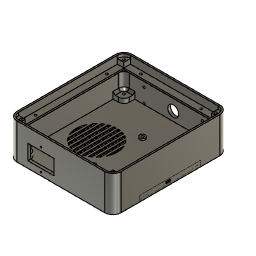
Solder Reflow Hot Plate Base (Autodesk Fusion 360 design; units mm, degrees)
Autodesk Fusion 360 part; units mm, degrees
note: some values were not read from the file. Chosen so that the rebuilt part matches the saved one: which bodies a step acts on; which face or edge a step refers to.
(part 1 of 2)
sketch "Base" plane through (0, 0, 0) normal (0, 0, 1) x (1, 0, 0) in component "Solder Reflow Hot Plate Base"
  line L0 (0, 0) -> (190, 0)
  line L1 (190, 0) -> (190, 210)
  line L2 (190, 210) -> (0, 210)
  line L3 (0, 210) -> (0, 0)
  dimension "d1" = 190
  dimension "d2" = 210
  constraint horizontal L0
  constraint vertical L1
  constraint horizontal L2
  constraint vertical L3
  constraint coincident L0.start L3.end
  measures "d1" distance of L0.start L0.end
  measures "d2" distance of L0.start L2.end
extrude "Extrude1" add sketch "Base" along normal blind 65 makes body 1 in component "Solder Reflow Hot Plate Base"
fillet "Fillet1" radius 15 4 edges at (0, 210, 32.5) (0, 0, 32.5) (190, 0, 32.5) (190, 210, 32.5) on bodies 1 in component "Solder Reflow Hot Plate Base"
shell "Shell1" thickness 5 removed faces 1 at (63.3333, 135, 65) on bodies 1 in component "Solder Reflow Hot Plate Base"
extrude "Extrude2" cut 1 faces at (65, 135, 5) along direction (0, 0, -1) blind 3 on bodies 1 bodies 1 in component "Solder Reflow Hot Plate Base"
sketch "Board Mount Split Sketch" plane through (0, 0, 2) normal (0, 0, 1) x (-1, 0, 0) in component "Solder Reflow Hot Plate Base"
  arc A0 (-185, -195) -> (-175, -205) centre (-175, -195) ccw
  line L0 (-175, -205) -> (-15, -205)
  arc A1 (-15, -205) -> (-5, -195) centre (-15, -195) ccw
  line L1 (-5, -195) -> (-5, -15)
  arc A2 (-5, -15) -> (-15, -5) centre (-15, -15) ccw
  line L2 (-15, -5) -> (-175, -5)
  arc A3 (-175, -5) -> (-185, -15) centre (-175, -15) ccw
  line L3 (-185, -15) -> (-185, -195)
  line L4 (-184.6, -15) -> (-184.6, -195)
  arc A4 (-184.6, -195) -> (-175, -204.6) centre (-175, -195) ccw
  line L5 (-175, -204.6) -> (-15, -204.6)
  arc A5 (-15, -204.6) -> (-5.4, -195) centre (-15, -195) ccw
  line L6 (-5.4, -195) -> (-5.4, -15)
  arc A6 (-5.4, -15) -> (-15, -5.4) centre (-15, -15) ccw
  line L7 (-15, -5.4) -> (-175, -5.4)
  arc A7 (-175, -5.4) -> (-184.6, -15) centre (-175, -15) ccw
  line L8 (-185, -15) -> (-185, -195)
  arc A8 (-185, -195) -> (-175, -205) centre (-175, -195) ccw
  line L9 (-175, -205) -> (-15, -205)
  arc A9 (-15, -205) -> (-5, -195) centre (-15, -195) ccw
  line L10 (-5, -195) -> (-5, -15)
  arc A10 (-5, -15) -> (-15, -5) centre (-15, -15) ccw
  line L11 (-15, -5) -> (-175, -5)
  arc A11 (-175, -5) -> (-185, -15) centre (-175, -15) ccw
  dimension "d10" = -0.4
  dimension "d11" = 0
  measures "d11" distance of L3
sketch "Sketch1" plane through (0, 0, 2) normal (0, 0, 1) x (-1, 0, 0)
  arc A0 (-185, -195) -> (-175, -205) centre (-175, -195) ccw
  line L0 (-175, -205) -> (-15, -205)
  arc A1 (-15, -205) -> (-5, -195) centre (-15, -195) ccw
  line L1 (-5, -195) -> (-5, -15)
  arc A2 (-5, -15) -> (-15, -5) centre (-15, -15) ccw
  line L2 (-15, -5) -> (-175, -5)
  arc A3 (-175, -5) -> (-185, -15) centre (-175, -15) ccw
  line L3 (-185, -15) -> (-185, -195)
  line L4 (-5, -195) -> (-5, -15)
  arc A4 (-5, -15) -> (-15, -5) centre (-15, -15) ccw
  line L5 (-15, -5) -> (-175, -5)
  arc A5 (-175, -5) -> (-185, -15) centre (-175, -15) ccw
  line L6 (-185, -15) -> (-185, -195)
  arc A6 (-185, -195) -> (-175, -205) centre (-175, -195) ccw
  line L7 (-175, -205) -> (-15, -205)
  arc A7 (-15, -205) -> (-5, -195) centre (-15, -195) ccw
  dimension "d12" = 0
  measures "d12" distance of L1
split "Split2" by curves path "Sketch1" along L4 A4 L5 A5 L6 A6 L7 A7 bodies 1 makes body 2 at (0, 135, 21.6667) in component "Solder Reflow Hot Plate Base"
sketch "Sketch2" plane through (0, 0, 2) normal (0, 0, 1) x (-1, 0, 0)
  arc A0 (-185, -195) -> (-175, -205) centre (-175, -195) ccw
  line L0 (-175, -205) -> (-15, -205)
  arc A1 (-15, -205) -> (-5, -195) centre (-15, -195) ccw
  line L1 (-5, -195) -> (-5, -15)
  arc A2 (-5, -15) -> (-15, -5) centre (-15, -15) ccw
  line L2 (-15, -5) -> (-175, -5)
  arc A3 (-175, -5) -> (-185, -15) centre (-175, -15) ccw
  line L3 (-185, -15) -> (-185, -195)
  line L4 (-5.4, -195) -> (-5.4, -15)
  arc A4 (-5.4, -15) -> (-15, -5.4) centre (-15, -15) ccw
  line L5 (-15, -5.4) -> (-175, -5.4)
  arc A5 (-175, -5.4) -> (-184.6, -15) centre (-175, -15) ccw
  line L6 (-184.6, -15) -> (-184.6, -195)
  arc A6 (-184.6, -195) -> (-175, -204.6) centre (-175, -195) ccw
  line L7 (-175, -204.6) -> (-15, -204.6)
  arc A7 (-15, -204.6) -> (-5.4, -195) centre (-15, -195) ccw
  dimension "d13" = -0.4
extrude "Extrude3" cut sketch "Sketch2" against normal up to surface (2 mm away) bodies 1 in component "Solder Reflow Hot Plate Base"
ref_plane "WorkPlane1" through (95, 105, 0) normal (0, 0, -1) x (-1, 0, 0) in component "Solder Reflow Hot Plate Base"
sketch "Sketch5" plane through (0, 0, 2) normal (0, 0, 1) x (-1, 0, 0) in component "Solder Reflow Hot Plate Base"
  line L0 (-15, -5.4) -> (-175, -5.4)
  arc A0 (-175, -5.4) -> (-184.6, -15) centre (-175, -15) ccw
  line L1 (-184.6, -15) -> (-184.6, -195)
  arc A1 (-184.6, -195) -> (-175, -204.6) centre (-175, -195) ccw
  line L2 (-175, -204.6) -> (-15, -204.6)
  arc A2 (-15, -204.6) -> (-5.4, -195) centre (-15, -195) ccw
  line L3 (-5.4, -195) -> (-5.4, -15)
  arc A3 (-5.4, -15) -> (-15, -5.4) centre (-15, -15) ccw
  line L4 (-184.6, -105) -> (-5.4, -105) construction
  line L5 (-184.6, -105) -> (-184.6, -50) construction
  line L6 (-184.6, -105) -> (-184.6, -160) construction
  line L7 (-184.6, -50) -> (-188.8, -50)
  line L8 (-184.6, -160) -> (-188.8, -160)
  line L9 (-188.8, -160) -> (-188.8, -50)
  line L10 (-184.6, -50) -> (-184.6, -160)
  dimension "d18" = 55
  dimension "d19" = 55
  dimension "d20" = 4.2
  dimension "d21" = 4.2
  constraint midpoint L1 L4.start
  constraint midpoint L3 L4.end
  constraint perpendicular L4 L5
  constraint perpendicular L4 L6
  constraint perpendicular L1 L7
  constraint perpendicular L1 L8
  measures "d18" distance of L4.start L5.end
  measures "d19" distance of L4.start L6.end
  measures "d20" distance of L5.end L7.end
  measures "d21" distance of L6.end L8.end
extrude "Extrude4" add sketch "Sketch5" against normal up to surface (2 mm away) contours L1 L7 L8 L9 L10 bodies 1 in component "Solder Reflow Hot Plate Base"
sketch "Sketch6" plane through (0, 0, 0) normal (0, 0, -1) x (1, 0, 0) in component "Solder Reflow Hot Plate Base"
  line L0 (175, -205) -> (15, -205)
  arc A0 (5, -195) -> (15, -205) centre (15, -195) ccw
  line L1 (5, -195) -> (5, -15)
  arc A1 (15, -5) -> (5, -15) centre (15, -15) ccw
  line L2 (15, -5) -> (175, -5)
  arc A2 (185, -15) -> (175, -5) centre (175, -15) ccw
  line L3 (185, -15) -> (185, -195)
  arc A3 (175, -205) -> (185, -195) centre (175, -195) ccw
  arc A4 (175, -210) -> (190, -195) centre (175, -195) ccw
  line L4 (190, -195) -> (190, -15)
  arc A5 (190, -15) -> (175, 0) centre (175, -15) ccw
  line L5 (175, 0) -> (15, 0)
  arc A6 (15, 0) -> (0, -15) centre (15, -15) ccw
  line L6 (0, -15) -> (0, -195)
  arc A7 (0, -195) -> (15, -210) centre (15, -195) ccw
  line L7 (15, -210) -> (175, -210)
  line L8 (190, -105) -> (189, -105) construction
  line L9 (189, -105) -> (189, -160.4)
  line L10 (189, -105) -> (189, -49.6)
  line L11 (189, -160.4) -> (185, -160.4)
  line L12 (189, -49.6) -> (185, -49.6)
  line L13 (185, -49.6) -> (185, -160.4)
  dimension "d27" = 55.4
  dimension "d28" = 55.4
  dimension "d31" = 1
  constraint midpoint L4 L8.start
  constraint perpendicular L4 L8
  constraint perpendicular L8 L9
  constraint perpendicular L8 L10
  constraint coincident L3 L11.end
  constraint perpendicular L3 L11
  constraint coincident L3 L12.end
  constraint perpendicular L3 L12
  measures "d27" distance of L8.end L9.end
  measures "d28" distance of L8.end L10.end
  measures "d31" distance of L4 L10
extrude "Extrude5" cut sketch "Sketch6" against normal blind 10 contours L3 L9 L10 L11 L12 L13 bodies 2 in component "Solder Reflow Hot Plate Base"
sketch "Sketch7" plane through (0, 0, 2) normal (0, 0, 1) x (-1, 0, 0) in component "Solder Reflow Hot Plate Base"
  line L0 (-15, -5.4) -> (-175, -5.4)
  arc A0 (-175, -5.4) -> (-184.6, -15) centre (-175, -15) ccw
  line L1 (-184.6, -15) -> (-184.6, -50)
  line L2 (-184.6, -50) -> (-188.8, -50)
  line L3 (-188.8, -50) -> (-188.8, -160)
  line L4 (-188.8, -160) -> (-184.6, -160)
  line L5 (-184.6, -160) -> (-184.6, -195)
  arc A1 (-184.6, -195) -> (-175, -204.6) centre (-175, -195) ccw
  line L6 (-175, -204.6) -> (-15, -204.6)
  arc A2 (-15, -204.6) -> (-5.4, -195) centre (-15, -195) ccw
  line L7 (-5.4, -195) -> (-5.4, -15)
  arc A3 (-5.4, -15) -> (-15, -5.4) centre (-15, -15) ccw
  line L8 (-188.8, -105) -> (-5.4, -105) construction
  line L9 (-184, -105) -> (-184, -60) construction
  line L10 (-184, -105) -> (-184, -150) construction
  circle A4 centre (-184, -60) radius 2.05
  circle A5 centre (-184, -150) radius 2.05
  line L11 (-94, -105) -> (-94, -60) construction
  line L12 (-94, -105) -> (-94, -150) construction
  circle A6 centre (-94, -60) radius 2.05
  circle A7 centre (-94, -150) radius 2.05
  circle A8 centre (-94, -150) radius 5
  circle A9 centre (-94, -60) radius 5
  line L13 (-184, -55) -> (-188.8, -55)
  line L14 (-184, -65) -> (-188.8, -65)
  arc A10 (-184, -65) -> (-184, -55) centre (-184, -60) ccw
  line L15 (-188.8, -55) -> (-188.8, -65)
  line L16 (-184, -145) -> (-188.8, -145)
  line L17 (-184, -155) -> (-188.8, -155)
  arc A11 (-184, -155) -> (-184, -145) centre (-184, -150) ccw
  line L18 (-188.8, -145) -> (-188.8, -155)
  dimension "d32" = 45
  dimension "d33" = 45
  dimension "d34" = 4.8
  dimension "d35" = 4.1
  dimension "d36" = 4.1
  dimension "d37" = 45
  dimension "d38" = 45
  dimension "d39" = 90
  dimension "d40" = 4.1
  dimension "d41" = 4.1
  dimension "d42" = 10
  dimension "d43" = 10
  dimension "d44" = 10
  dimension "d45" = 10
  constraint midpoint L3 L8.start
  constraint midpoint L7 L8.end
  constraint coincident L8 L9.start
  constraint perpendicular L8 L9
  constraint perpendicular L8 L10
  constraint coincident L9.end A4.centre
  constraint coincident L10.end A5.centre
  constraint coincident L8 L11.start
  constraint perpendicular L8 L11
  constraint perpendicular L8 L12
  constraint coincident L11.end A6.centre
  constraint coincident L12.end A7.centre
  constraint coincident L3 L13.end
  constraint tangent L13 A10
  constraint perpendicular L3 L13
  constraint coincident L9 L14.start
  constraint coincident L3 L14.end
  constraint tangent L14 A10
  constraint coincident L10 L16.start
  constraint coincident L3 L16.end
  constraint tangent L16 A11
  constraint coincident L3 L17.end
  constraint tangent L17 A11
  constraint perpendicular L3 L17
  measures "d32" distance of L9.start L9.end
  measures "d33" distance of L9.start L10.end
  measures "d34" distance of L3 L9
  measures "d35" diameter of A4
  measures "d36" diameter of A5
  measures "d37" distance of L11.start L11.end
  measures "d38" distance of L11.start L12.end
  measures "d39" distance of L9 L11
  measures "d40" diameter of A6
  measures "d41" diameter of A7
  measures "d42" diameter of A8
  measures "d43" diameter of A9
  measures "d44" diameter of A10
  measures "d45" diameter of A11
extrude "Extrude6" add sketch "Sketch7" along normal blind 3 contours L3 L13 L14 A10 L15 | L3 L16 L17 A11 L18 | A8 | A9 bodies 1 in component "Solder Reflow Hot Plate Base"
extrude "Extrude7" cut 4 faces at (94.4261, 150.7379, 2) (184.6757, 149.8982, 2) (93.7504, 60.6361, 2) (183.4991, 59.1324, 2) along direction (0, 0, 1) up to surface end surface through (0, 0, 0) normal (0, 0, -1) offset 0 on bodies 1 bodies 1 in component "Solder Reflow Hot Plate Base"
sketch "Sketch8" plane through (190, 0, 0) normal (1, 0, 0) x (0, 1, 0) in component "Solder Reflow Hot Plate Base"
  line L0 (195, 0) -> (195, 65)
  line L1 (195, 65) -> (15, 65)
  line L2 (15, 65) -> (15, 0)
  line L3 (15, 0) -> (195, 0)
  line L4 (105, 0) -> (105, 65) construction
  line L5 (100.8, 0) -> (100.8, 65) construction
  line L6 (55, 5) -> (65, 5) construction
  line L7 (145, 5) -> (155, 5) construction
  line L8 (55, 5) -> (155, 5) construction
  line L9 (55, 4.8) -> (155, 4.8) construction
  line L10 (96.8, 0) -> (96.8, 65) construction
  line L11 (104.8, 0) -> (104.8, 65) construction
  line L12 (15, 8.2) -> (195, 8.2) construction
  line L13 (96.8, 8.2) -> (104.8, 8.2)
  line L14 (104.8, 8.2) -> (104.8, 4.8)
  line L15 (104.8, 4.8) -> (96.8, 4.8)
  line L16 (96.8, 4.8) -> (96.8, 8.2)
  dimension "d50" = 4.2
  dimension "d51" = 0.2
  dimension "d52" = 4
  dimension "d53" = 4
  dimension "d54" = 3.4
  constraint midpoint L3 L4.start
  constraint midpoint L1 L4.end
  constraint coincident L3 L5.start
  constraint coincident L1 L5.end
  constraint perpendicular L1 L5
  constraint coincident L6.start L8.start
  constraint coincident L7.end L8.end
  constraint parallel L8 L9
  constraint coincident L3 L10.start
  constraint coincident L1 L10.end
  constraint perpendicular L1 L10
  constraint coincident L3 L11.start
  constraint coincident L1 L11.end
  constraint perpendicular L1 L11
  constraint coincident L2 L12.start
  constraint coincident L0 L12.end
  constraint perpendicular L0 L12
  constraint horizontal L13
  constraint vertical L14
  constraint horizontal L15
  constraint vertical L16
  constraint coincident L9 L14.end
  constraint coincident L11 L14.end
  constraint coincident L12 L13.start
  constraint coincident L10 L13.start
  measures "d50" distance of L4 L5
  measures "d51" distance of L8 L9
  measures "d52" distance of L5 L10
  measures "d53" distance of L5 L11
  measures "d54" distance of L9 L12
extrude "Extrude8" cut sketch "Sketch8" against normal up to surface (1 mm away) contours L13 L14 L15 L16 bodies 2 in component "Solder Reflow Hot Plate Base"
chamfer "Chamfer1" distance 0.5 angle 45 2 edges at (189.5, 104.8, 4.8) (189.5, 96.8, 4.8) on bodies 2 in component "Solder Reflow Hot Plate Base"
ref_plane "WorkPlane2" through (95, 105, 2) normal (0, 0, -1) x (-1, 0, 0) in component "Solder Reflow Hot Plate Base"
sketch "Sketch9" plane through (95, 105, 2) normal (0, 0, -1) x (1, 0, 0) in component "Solder Reflow Hot Plate Base"
  line L0 (90, -90) -> (90, 90) construction
  arc A0 (90, 90) -> (80, 100) centre (80, 90) ccw construction
  line L1 (80, 100) -> (-80, 100) construction
  arc A1 (-80, 100) -> (-90, 90) centre (-80, 90) ccw construction
  line L2 (-90, 90) -> (-90, -90) construction
  arc A2 (-90, -90) -> (-80, -100) centre (-80, -90) ccw construction
  line L3 (-80, -100) -> (80, -100) construction
  arc A3 (80, -100) -> (90, -90) centre (80, -90) ccw construction
  arc A4 (80, -100) -> (90, -90) centre (80, -90) ccw construction
  line L4 (90, -90) -> (90, 90) construction
  arc A5 (90, 90) -> (80, 100) centre (80, 90) ccw construction
  line L5 (80, 100) -> (-80, 100) construction
  arc A6 (-80, 100) -> (-90, 90) centre (-80, 90) ccw construction
  line L6 (-90, 90) -> (-90, -90) construction
  arc A7 (-90, -90) -> (-80, -100) centre (-80, -90) ccw construction
  line L7 (-80, -100) -> (80, -100) construction
  arc A8 (80, -105) -> (95, -90) centre (80, -90) ccw construction
  line L8 (80, -105) -> (-80, -105) construction
  arc A9 (-95, -90) -> (-80, -105) centre (-80, -90) ccw construction
  line L9 (-95, -90) -> (-95, 90) construction
  arc A10 (-80, 105) -> (-95, 90) centre (-80, 90) ccw construction
  line L10 (-80, 105) -> (80, 105) construction
  arc A11 (95, 90) -> (80, 105) centre (80, 90) ccw construction
  line L11 (95, 90) -> (95, -90) construction
  line L12 (80, 100) -> (80, -100) construction
  line L13 (90, -90) -> (-90, -90) construction
  line L14 (-80, -100) -> (-80, 100) construction
  line L15 (90, 90) -> (-90, 90) construction
  circle A12 centre (80, 90) radius 2.05
  line L16 (80, 80) -> (90, 80)
  line L17 (70, 90) -> (70, 100)
  line L18 (70, 100) -> (80, 100)
  line L19 (90, 80) -> (90, 90)
  arc A13 (70, 90) -> (80, 80) centre (80, 90) ccw
  arc A14 (90, 90) -> (80, 100) centre (80, 90) ccw
  line L20 (0, 100) -> (0, -100) construction
  line L21 (90, 0) -> (-90, 0) construction
  line L22 (-70, 100) -> (-80, 100)
  line L23 (-70, 90) -> (-70, 100)
  arc A15 (-80, 80) -> (-70, 90) centre (-80, 90) ccw
  line L24 (-80, 80) -> (-90, 80)
  line L25 (-90, 80) -> (-90, 90)
  arc A16 (-80, 100) -> (-90, 90) centre (-80, 90) ccw
  circle A17 centre (-80, 90) radius 2.05
  line L26 (80, -80) -> (90, -80)
  line L27 (90, -80) -> (90, -90)
  arc A18 (80, -100) -> (90, -90) centre (80, -90) ccw
  line L28 (70, -100) -> (80, -100)
  line L29 (70, -90) -> (70, -100)
  arc A19 (80, -80) -> (70, -90) centre (80, -90) ccw
  circle A20 centre (80, -90) radius 2.05
  line L30 (-70, -90) -> (-70, -100)
  line L31 (-70, -100) -> (-80, -100)
  arc A21 (-90, -90) -> (-80, -100) centre (-80, -90) ccw
  line L32 (-90, -80) -> (-90, -90)
  line L33 (-80, -80) -> (-90, -80)
  arc A22 (-70, -90) -> (-80, -80) centre (-80, -90) ccw
  circle A23 centre (-80, -90) radius 2.05
  dimension "d60" = 4.1
  constraint coincident A0.end L1.start
  constraint coincident L3.end A3.start
  constraint coincident L0.start A3.end
  constraint coincident L2.end A2.start
  constraint coincident A2.end L3.start
  constraint coincident L1.end A1.start
  constraint coincident L0.end A0.start
  constraint coincident A1.end L2.start
  constraint concentric A0 A12
  constraint concentric A5 A13
  constraint coincident A0.end A13
  constraint coincident L12 L16.start
  constraint coincident L4 L16.end
  constraint tangent L16 A13
  constraint coincident L15 L17.start
  constraint coincident L1 L17.end
  constraint tangent L17 A13
  constraint concentric A13 A14
  constraint midpoint L5 L20.start
  constraint midpoint L3 L20.end
  constraint midpoint L0 L21.start
  constraint midpoint L6 L21.end
  constraint symmetric L0.end L20 A1.end
  constraint symmetric A0.end L20 L1.end
  constraint symmetric A12 L20 A17
  constraint symmetric L16.start L20 A15.start
  constraint symmetric L16.end L20 L24.end
  constraint symmetric L17.start L20 L23.start
  constraint symmetric L17.end L20 L22.start
  constraint symmetric A13 L20 A15
  constraint symmetric A14 L20 A16
  constraint symmetric L0.end L21 L0.start
  constraint symmetric A0.end L21 L3.end
  constraint symmetric A12 L21 A20
  constraint symmetric L16.start L21 L26.start
  constraint symmetric L16.end L21 L26.end
  constraint symmetric L17.start L21 L29.start
  constraint symmetric L17.end L21 L28.start
  constraint symmetric A13 L21 A19
  constraint symmetric A14 L21 A18
  constraint symmetric L21 L22.start L30.end
  constraint symmetric L21 L1.end A2.end
  constraint symmetric L21 L23.start L30.start
  constraint symmetric L21 A15.start L33.start
  constraint symmetric L21 A15 A22
  constraint symmetric L21 L24.end L32.start
  constraint symmetric L21 A1.end L2.end
  constraint symmetric L21 A16 A21
  constraint symmetric L21 A17 A23
  measures "d60" diameter of A12
extrude "Extrude9" add sketch "Sketch9" against normal blind 8 bodies 2 in component "Solder Reflow Hot Plate Base"
chamfer "Chamfer2" distance 4 angle 45 12 edges at (182.0711, 7.9289, 10) (170, 5, 10) (185, 20, 10) (20, 5, 10) (7.9289, 7.9289, 10) (5, 20, 10) (20, 205, 10) (5, 190, 10) (7.9289, 202.0711, 10) (170, 205, 10) (182.0711, 202.0711, 10) (185, 190, 10) on bodies 2 in component "Solder Reflow Hot Plate Base"
sketch "Sketch10" plane through (0, 0, 0) normal (0, 0, -1) x (1, 0, 0) in component "Solder Reflow Hot Plate Base"
  circle A0 centre (94, -60) radius 2.05
  circle A1 centre (94, -150) radius 2.05
  circle A2 centre (184, -150) radius 2.05
  circle A3 centre (184, -60) radius 2.05
  line L0 (175, -5.4) -> (15, -5.4)
  arc A4 (15, -5.4) -> (5.4, -15) centre (15, -15) ccw
  line L1 (5.4, -15) -> (5.4, -195)
  arc A5 (5.4, -195) -> (15, -204.6) centre (15, -195) ccw
  line L2 (15, -204.6) -> (175, -204.6)
  arc A6 (175, -204.6) -> (184.6, -195) centre (175, -195) ccw
  line L3 (184.6, -195) -> (184.6, -160)
  line L4 (184.6, -160) -> (188.8, -160)
  line L5 (188.8, -160) -> (188.8, -50)
  line L6 (188.8, -50) -> (184.6, -50)
  line L7 (184.6, -50) -> (184.6, -15)
  arc A7 (184.6, -15) -> (175, -5.4) centre (175, -15) ccw
  circle A8 centre (175, -15) radius 2.05
  circle A9 centre (15, -15) radius 2.05
  circle A10 centre (15, -195) radius 2.05
  circle A11 centre (175, -195) radius 2.05
  circle A12 centre (15, -195) radius 1.9
  circle A13 centre (175, -195) radius 1.9
  circle A14 centre (175, -15) radius 1.9
  circle A15 centre (15, -15) radius 1.9
  dimension "d71" = 3.8
  dimension "d72" = 3.8
  dimension "d73" = 3.8
  dimension "d74" = 3.8
  constraint concentric A10 A12
  constraint concentric A11 A13
  constraint concentric A7 A14
  constraint concentric A9 A15
  measures "d71" diameter of A12
  measures "d72" diameter of A13
  measures "d73" diameter of A14
  measures "d74" diameter of A15
extrude "Extrude10" cut sketch "Sketch10" against normal up to surface (2 mm away) contours A12 | A13 | A14 | A15 bodies 1 in component "Solder Reflow Hot Plate Base"
ref_plane "WorkPlane3" through (95, 105, 31) normal (0, 0, -1) x (-1, 0, 0) in component "Solder Reflow Hot Plate Base"
ref_plane "WorkPlane4" through (95, 105, 60) normal (0, 0, 1) x (1, 0, 0) in component "Solder Reflow Hot Plate Base"
ref_plane "WorkPlane5" through (95, 105, 51) normal (0, 0, 1) x (1, 0, 0) in component "Solder Reflow Hot Plate Base"
sketch "Sketch11" plane through (0, 0, 65) normal (0, 0, 1) x (-1, 0, 0) in component "Solder Reflow Hot Plate Base"
  arc A0 (-185, -195) -> (-175, -205) centre (-175, -195) ccw
  line L0 (-185, -195) -> (-185, -15)
  arc A1 (-175, -5) -> (-185, -15) centre (-175, -15) ccw
  line L1 (-175, -5) -> (-15, -5)
  arc A2 (-5, -15) -> (-15, -5) centre (-15, -15) ccw
  line L2 (-5, -15) -> (-5, -195)
  arc A3 (-15, -205) -> (-5, -195) centre (-15, -195) ccw
  line L3 (-15, -205) -> (-175, -205)
  arc A4 (-190, -195) -> (-175, -210) centre (-175, -195) ccw
  line L4 (-175, -210) -> (-15, -210)
  arc A5 (-15, -210) -> (0, -195) centre (-15, -195) ccw
  line L5 (0, -195) -> (0, -15)
  arc A6 (0, -15) -> (-15, 0) centre (-15, -15) ccw
  line L6 (-15, 0) -> (-175, 0)
  arc A7 (-175, 0) -> (-190, -15) centre (-175, -15) ccw
  line L7 (-190, -15) -> (-190, -195)
  arc A8 (-3, -15) -> (-15, -3) centre (-15, -15) ccw
  line L8 (-175, -3) -> (-15, -3)
  arc A9 (-175, -3) -> (-187, -15) centre (-175, -15) ccw
  line L9 (-187, -195) -> (-187, -15)
  arc A10 (-187, -195) -> (-175, -207) centre (-175, -195) ccw
  line L10 (-15, -207) -> (-175, -207)
  arc A11 (-15, -207) -> (-3, -195) centre (-15, -195) ccw
  line L11 (-3, -15) -> (-3, -195)
  arc A12 (-5, -15) -> (-15, -5) centre (-15, -15) ccw
  line L12 (-175, -5) -> (-15, -5)
  arc A13 (-175, -5) -> (-185, -15) centre (-175, -15) ccw
  line L13 (-185, -195) -> (-185, -15)
  arc A14 (-185, -195) -> (-175, -205) centre (-175, -195) ccw
  line L14 (-15, -205) -> (-175, -205)
  arc A15 (-15, -205) -> (-5, -195) centre (-15, -195) ccw
  line L15 (-5, -15) -> (-5, -195)
  dimension "d80" = -2
  dimension "d81" = 0
extrude "Extrude11" cut sketch "Sketch11" against normal up to surface (14 mm away) contours A8 L8 A9 L9 A10 L10 A11 L11 bodies 2 in component "Solder Reflow Hot Plate Base"
sketch "Sketch12" plane through (0, 0, 51) normal (0, 0, 1) x (-1, 0, 0) in component "Solder Reflow Hot Plate Base"
  line L0 (-175, -5) -> (-15, -5)
  arc A0 (-5, -15) -> (-15, -5) centre (-15, -15) ccw
  line L1 (-5, -15) -> (-5, -195)
  arc A1 (-15, -205) -> (-5, -195) centre (-15, -195) ccw
  line L2 (-15, -205) -> (-175, -205)
  arc A2 (-185, -195) -> (-175, -205) centre (-175, -195) ccw
  line L3 (-185, -195) -> (-185, -15)
  arc A3 (-175, -5) -> (-185, -15) centre (-175, -15) ccw
  line L4 (-187, -15) -> (-187, -195)
  arc A4 (-187, -195) -> (-175, -207) centre (-175, -195) ccw
  line L5 (-175, -207) -> (-15, -207)
  arc A5 (-15, -207) -> (-3, -195) centre (-15, -195) ccw
  line L6 (-3, -195) -> (-3, -15)
  arc A6 (-3, -15) -> (-15, -3) centre (-15, -15) ccw
  line L7 (-15, -3) -> (-175, -3)
  arc A7 (-175, -3) -> (-187, -15) centre (-175, -15) ccw
  line L8 (-185, -15) -> (-5, -15) construction
  line L9 (-175, -5) -> (-175, -205) construction
  line L10 (-175, -15) -> (-15, -15)
  line L11 (-175, -195) -> (-175, -15)
  line L12 (-15, -195) -> (-175, -195)
  line L13 (-15, -15) -> (-15, -195)
  dimension "d84" = 10
  constraint coincident L3.end A3.end
  constraint coincident A0.start L1.start
  constraint coincident L0.start A3.start
  constraint coincident L2.end A2.end
extrude "Extrude12" add sketch "Sketch12" against normal blind 3 contours L0 A0 L1 A1 L2 A2 L3 A3 bodies 2 in component "Solder Reflow Hot Plate Base"
chamfer "Chamfer3" distance 9.8 angle 45 8 edges at (185, 105, 48) (182.0711, 202.0711, 48) (95, 205, 48) (7.9289, 202.0711, 48) (5, 105, 48) (7.9289, 7.9289, 48) (95, 5, 48) (182.0711, 7.9289, 48) on bodies 2 in component "Solder Reflow Hot Plate Base"
sketch "Sketch13" plane through (0, 0, 51) normal (0, 0, 1) x (-1, 0, 0) in component "Solder Reflow Hot Plate Base"
  line L0 (-175, -15) -> (-15, -15)
  line L1 (-15, -15) -> (-15, -195)
  line L2 (-15, -195) -> (-175, -195)
  line L3 (-175, -195) -> (-175, -15)
  line L4 (-187, -15) -> (-187, -195)
  arc A0 (-187, -195) -> (-175, -207) centre (-175, -195) ccw
  line L5 (-175, -207) -> (-15, -207)
  arc A1 (-15, -207) -> (-3, -195) centre (-15, -195) ccw
  line L6 (-3, -195) -> (-3, -15)
  arc A2 (-3, -15) -> (-15, -3) centre (-15, -15) ccw
  line L7 (-15, -3) -> (-175, -3)
  arc A3 (-175, -3) -> (-187, -15) centre (-175, -15) ccw
  line L8 (-187, -15) -> (-3, -15) construction
  line L9 (-175, -3) -> (-175, -207) construction
  line L10 (-186.619, -12) -> (-3.381, -12) construction
  line L11 (-178, -3.381) -> (-178, -206.619) construction
  circle A4 centre (-178, -12) radius 2.05
  line L12 (-95, -3) -> (-95, -207) construction
  line L13 (-187, -105) -> (-3, -105) construction
  circle A5 centre (-12, -12) radius 2.05
  circle A6 centre (-12, -198) radius 2.05
  circle A7 centre (-178, -198) radius 2.05
  dimension "d88" = 3
  dimension "d89" = 3
  dimension "d90" = 4.1
  constraint coincident L4.start A3.end
  constraint coincident L6.end A2.start
  constraint coincident L7.end A3.start
  constraint coincident A0.end L5.start
  constraint horizontal L10
  constraint coincident A3 L10.start
  constraint coincident A2 L10.end
  constraint vertical L11
  constraint coincident A3 L11.start
  constraint coincident A0 L11.end
  constraint coincident L11 A4.centre
  constraint coincident L10 A4.centre
  constraint midpoint L7 L12.start
  constraint midpoint L5 L12.end
  constraint midpoint L4 L13.start
  constraint midpoint L6 L13.end
  constraint symmetric A4 L12 A5
  constraint symmetric A4 L13 A7
  constraint symmetric L13 A5 A6
  measures "d88" distance of L8 L10
  measures "d89" distance of L9 L11
  measures "d90" diameter of A4
sketch "Sketch15" plane through (0, 0, 51) normal (0, 0, 1) x (-1, 0, 0) in component "Solder Reflow Hot Plate Base"
  line L0 (-175, -15) -> (-15, -15)
  line L1 (-15, -15) -> (-15, -195)
  line L2 (-15, -195) -> (-175, -195)
  line L3 (-175, -195) -> (-175, -15)
  line L4 (-187, -15) -> (-187, -195)
  arc A0 (-187, -195) -> (-175, -207) centre (-175, -195) ccw
  line L5 (-175, -207) -> (-15, -207)
  arc A1 (-15, -207) -> (-3, -195) centre (-15, -195) ccw
  line L6 (-3, -195) -> (-3, -15)
  arc A2 (-3, -15) -> (-15, -3) centre (-15, -15) ccw
  line L7 (-15, -3) -> (-175, -3)
  arc A3 (-175, -3) -> (-187, -15) centre (-175, -15) ccw
  line L8 (-165, -15) -> (-165, -5)
  line L9 (-175, -25) -> (-185, -25)
  arc A4 (-175, -3) -> (-187, -15) centre (-175, -15) ccw
  line L10 (-95, -3) -> (-95, -207) construction
  line L11 (-187, -105) -> (-3, -105) construction
  line L12 (-175, -15) -> (-175, -14)
  line L13 (-175, -14) -> (-175, -3)
  line L14 (-175, -15) -> (-187, -15)
  line L15 (-15, -15) -> (-3, -15)
  line L16 (-15, -195) -> (-3, -195)
  line L17 (-175, -195) -> (-187, -195)
  line L18 (-15, -15) -> (-15, -3)
  line L19 (-15, -195) -> (-15, -207)
  line L20 (-175, -195) -> (-175, -207)
  circle A5 centre (-179, -11) radius 2.05
  circle A6 centre (-11, -11) radius 2.05
  circle A7 centre (-11, -199) radius 2.05
  circle A8 centre (-179, -199) radius 2.05
  dimension "d97" = 4.1
  dimension "d98" = 4
  dimension "d99" = 4
  constraint midpoint L7 L10.start
  constraint midpoint L5 L10.end
  constraint midpoint L4 L11.start
  constraint midpoint L6 L11.end
  constraint coincident L0.start L3.end
  constraint perpendicular L0 L12
  constraint coincident L7.end A3.start
  constraint perpendicular L7 L13
  constraint coincident L4.start A3.end
  constraint symmetric L10 L0.start L0.end
  constraint symmetric L10 L4.start L6.end
  constraint symmetric L11 L0.start L2.end
  constraint symmetric L11 L4.start L4.end
  constraint symmetric L11 L0.end L1.end
  constraint symmetric L11 L6.end A1.end
  constraint coincident A2.end L7.start
  constraint coincident L5.end A1.start
  constraint coincident A0.end L5.start
  constraint symmetric L10 A5 A6
  constraint symmetric L11 A5 A8
  constraint symmetric L11 A6 A7
  measures "d97" diameter of A5
  measures "d98" distance of L13 A5.centre
  measures "d99" distance of L14 A5.centre
extrude "Extrude16" add sketch "Sketch15" along normal blind 9 contours A3 A4 L12 L13 L14 | A2 L15 L18 | A0 L17 L20 | A1 L16 L19 bodies 2 in component "Solder Reflow Hot Plate Base"
sketch "Sketch16" plane through (0, 0, 0) normal (0, -1, 0) x (1, 0, 0) in component "Solder Reflow Hot Plate Base"
  line L0 (175, 0) -> (175, 65)
  line L1 (175, 65) -> (15, 65)
  line L2 (15, 65) -> (15, 0)
  line L3 (15, 0) -> (175, 0)
  line L4 (35, 39.5) -> (82.5, 39.5)
  line L5 (82.5, 39.5) -> (82.5, 12)
  line L6 (82.5, 12) -> (35, 12)
  line L7 (35, 12) -> (35, 39.5)
  line L8 (58.75, 39.5) -> (58.75, 45.5) construction
  line L9 (58.75, 12) -> (58.75, 6) construction
  circle A0 centre (58.75, 45.5) radius 1.4
  circle A1 centre (58.75, 6) radius 1.4
  line L10 (58.75, 39.5) -> (58.75, 12) construction
  line L11 (88.75, 39.5) -> (88.75, 12) construction
  line L12 (28.75, 39.5) -> (28.75, 12) construction
  dimension "d102" = 47.5
  dimension "d103" = 27.5
  dimension "d104" = 6
  dimension "d105" = 6
  dimension "d106" = 2.8
  dimension "d107" = 2.8
  dimension "d109" = 30
  dimension "d111" = 30
  dimension "d112" = 20
  dimension "d113" = 12
  constraint horizontal L4
  constraint vertical L5
  constraint horizontal L6
  constraint vertical L7
  constraint midpoint L4 L8.start
  constraint perpendicular L4 L8
  constraint midpoint L6 L9.start
  constraint perpendicular L6 L9
  constraint coincident L8.end A0.centre
  constraint coincident L9.end A1.centre
  constraint perpendicular L6 L11
  constraint perpendicular L6 L12
  measures "d102" distance of L4.start L4.end
  measures "d103" distance of L4.start L6.end
  measures "d104" distance of L8.start L8.end
  measures "d105" distance of L9.start L9.end
  measures "d106" diameter of A0
  measures "d107" diameter of A1
  measures "d109" distance of L10 L11
  measures "d111" distance of L10 L12
  measures "d112" distance of L2 L7
  measures "d113" distance of L3 L6
extrude "Extrude17" cut sketch "Sketch16" against normal blind 15 contours L4 L5 L6 L7 | A0 | A1 bodies 2 in component "Solder Reflow Hot Plate Base"
sketch "Sketch17" plane through (0, 0, 51) normal (0, 0, 1) x (-1, 0, 0) in component "Solder Reflow Hot Plate Base"
  line L0 (-175, -3) -> (-175, -15)
  line L1 (-175, -15) -> (-15, -15)
  line L2 (-15, -15) -> (-15, -3)
  line L3 (-15, -3) -> (-175, -3)
  line L4 (-35, 0) -> (-35, -6.3) construction
  line L5 (-82.5, 0) -> (-82.5, -6.3) construction
  line L6 (-35, 0) -> (-35, -15) construction
  line L7 (-82.5, 0) -> (-82.5, -15) construction
  line L8 (-82.5, -15) -> (-35, -15)
  line L9 (-35, -15) -> (-35, -3)
  line L10 (-35, -3) -> (-82.5, -3)
  line L11 (-82.5, -3) -> (-82.5, -15)
  constraint coincident L4.start L6.start
  constraint coincident L1 L6.end
  constraint perpendicular L1 L6
  constraint coincident L5.start L7.start
  constraint coincident L1 L7.end
  constraint perpendicular L1 L7
  constraint horizontal L8
  constraint vertical L9
  constraint horizontal L10
  constraint vertical L11
  constraint coincident L6 L9.end
extrude "Extrude19" cut sketch "Sketch17" against normal up to surface (11.5 mm away) contours L1 L3 L8 L9 L10 L11 bodies 2 in component "Solder Reflow Hot Plate Base"
ref_plane "WorkPlane6" through (95, 105, 32.5) normal (1, 0, 0) x (0, 1, 0) in component "Solder Reflow Hot Plate Base"
sketch "Sketch19" plane through (0, 0, 2) normal (0, 0, 1) x (-1, 0, 0) in component "Solder Reflow Hot Plate Base"
  circle A0 centre (-175, -15) radius 1.9
  circle A1 centre (-15, -195) radius 1.9
  circle A2 centre (-15, -15) radius 1.9
  circle A3 centre (-175, -195) radius 1.9
  line L0 (-188.8, -145) -> (-184, -145)
  arc A4 (-184, -155) -> (-184, -145) centre (-184, -150) ccw
  line L1 (-184, -155) -> (-188.8, -155)
  line L2 (-188.8, -155) -> (-188.8, -160)
  line L3 (-188.8, -160) -> (-184.6, -160)
  line L4 (-184.6, -160) -> (-184.6, -195)
  arc A5 (-184.6, -195) -> (-175, -204.6) centre (-175, -195) ccw
  line L5 (-175, -204.6) -> (-15, -204.6)
  arc A6 (-15, -204.6) -> (-5.4, -195) centre (-15, -195) ccw
  line L6 (-5.4, -195) -> (-5.4, -15)
  arc A7 (-5.4, -15) -> (-15, -5.4) centre (-15, -15) ccw
  line L7 (-15, -5.4) -> (-175, -5.4)
  arc A8 (-175, -5.4) -> (-184.6, -15) centre (-175, -15) ccw
  line L8 (-184.6, -15) -> (-184.6, -50)
  line L9 (-184.6, -50) -> (-188.8, -50)
  line L10 (-188.8, -50) -> (-188.8, -55)
  line L11 (-188.8, -55) -> (-184, -55)
  arc A9 (-184, -65) -> (-184, -55) centre (-184, -60) ccw
  line L12 (-184, -65) -> (-188.8, -65)
  line L13 (-188.8, -65) -> (-188.8, -145)
  circle A10 centre (-94, -60) radius 5
  circle A11 centre (-94, -150) radius 5
  line L14 (-184, -60) -> (-94, -60) construction
  line L15 (-184, -150) -> (-94, -150) construction
  line L16 (-188.8, -105) -> (-5.4, -105) construction
  line L17 (-57.4, -67.5534) -> (-57.4, -142.4466)
  line L18 (-53.4, -142.4466) -> (-53.4, -67.5534)
  line L19 (-89.4, -89.1807) -> (-89.4, -120.8193)
  line L20 (-85.4, -127.5) -> (-85.4, -82.5)
  line L21 (-81.4, -77.9769) -> (-81.4, -132.0231)
  line L22 (-77.4, -135.3686) -> (-77.4, -74.6314)
  line L23 (-73.4, -72.1024) -> (-73.4, -137.8976)
  line L24 (-69.4, -139.7886) -> (-69.4, -70.2114)
  line L25 (-65.4, -68.8579) -> (-65.4, -141.1421)
  line L26 (-61.4, -142.0169) -> (-61.4, -67.9831)
  line L27 (-49.4, -67.9831) -> (-49.4, -142.0169)
  line L28 (-45.4, -141.1421) -> (-45.4, -68.8579)
  line L29 (-41.4, -70.2114) -> (-41.4, -139.7886)
  line L30 (-37.4, -137.8976) -> (-37.4, -72.1024)
  line L31 (-33.4, -74.6314) -> (-33.4, -135.3686)
  line L32 (-29.4, -132.0231) -> (-29.4, -77.9769)
  line L33 (-25.4, -82.5) -> (-25.4, -127.5)
  line L34 (-21.4, -120.8193) -> (-21.4, -89.1807)
  arc A12 (-89.4, -89.1807) -> (-89.4, -120.8193) centre (-55.4, -105) ccw
  arc A13 (-81.4, -77.9769) -> (-85.4, -82.5) centre (-55.4, -105) ccw
  arc A14 (-85.4, -127.5) -> (-81.4, -132.0231) centre (-55.4, -105) ccw
  arc A15 (-73.4, -72.1024) -> (-77.4, -74.6314) centre (-55.4, -105) ccw
  arc A16 (-77.4, -135.3686) -> (-73.4, -137.8976) centre (-55.4, -105) ccw
  arc A17 (-65.4, -68.8579) -> (-69.4, -70.2114) centre (-55.4, -105) ccw
  arc A18 (-69.4, -139.7886) -> (-65.4, -141.1421) centre (-55.4, -105) ccw
  arc A19 (-61.4, -142.0169) -> (-57.4, -142.4466) centre (-55.4, -105) ccw
  arc A20 (-57.4, -67.5534) -> (-61.4, -67.9831) centre (-55.4, -105) ccw
  arc A21 (-53.4, -142.4466) -> (-49.4, -142.0169) centre (-55.4, -105) ccw
  arc A22 (-49.4, -67.9831) -> (-53.4, -67.5534) centre (-55.4, -105) ccw
  arc A23 (-41.4, -70.2114) -> (-45.4, -68.8579) centre (-55.4, -105) ccw
  arc A24 (-45.4, -141.1421) -> (-41.4, -139.7886) centre (-55.4, -105) ccw
  arc A25 (-37.4, -137.8976) -> (-33.4, -135.3686) centre (-55.4, -105) ccw
  arc A26 (-33.4, -74.6314) -> (-37.4, -72.1024) centre (-55.4, -105) ccw
  arc A27 (-25.4, -82.5) -> (-29.4, -77.9769) centre (-55.4, -105) ccw
  arc A28 (-29.4, -132.0231) -> (-25.4, -127.5) centre (-55.4, -105) ccw
  arc A29 (-21.4, -120.8193) -> (-21.4, -89.1807) centre (-55.4, -105) ccw
  point P0 (-55.4, -105)
  dimension "d260" = 75
  dimension "d261" = 50
  constraint coincident A9.centre L14.start
  constraint coincident A10.centre L14.end
  constraint coincident A4.centre L15.start
  constraint coincident A11.centre L15.end
  constraint midpoint L13 L16.start
  constraint midpoint L6 L16.end
  constraint coincident L16 P0
  constraint parallel L17 L18
  constraint coincident P0 A12.centre
  constraint coincident L22.start A14
  constraint coincident L23.end A14
  constraint coincident L24.start A14
  constraint coincident L25.end A14
  constraint coincident L26.start A14
  constraint coincident L17.end A14
  constraint coincident L18.start A14
  constraint coincident L27.end A14
  constraint coincident L28.start A14
  constraint coincident L34.start A14
  constraint coincident L33.end A14
  constraint coincident L32.start A14
  constraint coincident L31.end A14
  constraint coincident L30.start A14
  constraint coincident L29.end A14
  constraint coincident L19.start A14
  constraint coincident L21.start A14
  constraint coincident L23.start A14
  constraint coincident L24.end A14
  constraint coincident L25.start A14
  constraint coincident L26.end A14
  constraint coincident L17.start A14
  constraint coincident L18.end A14
  constraint coincident L27.start A14
  constraint coincident L28.end A14
  constraint coincident L29.start A14
  constraint coincident L30.end A14
  constraint coincident L31.start A14
  constraint coincident L32.end A14
  constraint coincident L33.start A14
  constraint coincident L34.end A14
  constraint concentric A12 A14
  constraint concentric A13 A14
  constraint concentric A14 A16
  constraint concentric A15 A16
  constraint concentric A16 A18
  constraint concentric A17 A18
  constraint concentric A18 A19
  constraint concentric A19 A21
  constraint concentric A20 A21
  constraint concentric A21 A24
  constraint concentric A22 A24
  constraint concentric A23 A24
  constraint concentric A24 A25
  constraint concentric A25 A28
  constraint concentric A26 A28
  constraint concentric A27 A28
  constraint concentric A28 A29
  measures "d260" diameter of A14
  measures "d261" distance of L6 P0
extrude "Extrude21" cut sketch "Sketch19" against normal up to surface (2 mm away) contours L17 L26 A19 A20 | L18 L27 A21 A22 | L19 A12 | L20 L21 A13 A14 | L22 L23 A15 A16 | L24 L25 A17 A18 | L28 L29 A23 A24 | L30 L31 A25 A26 | L32 L33 A27 A28 | L34 A29 bodies 1 in component "Solder Reflow Hot Plate Base"
sketch "Sketch20" plane through (0, 210, 0) normal (0, 1, 0) x (-1, 0, 0) in component "Solder Reflow Hot Plate Base"
  line L0 (-175, 65) -> (-175, 0)
  line L1 (-175, 0) -> (-15, 0)
  line L2 (-15, 0) -> (-15, 65)
  line L3 (-15, 65) -> (-175, 65)
  line L4 (-95, 65) -> (-95, 0) construction
  line L5 (-95, 35) -> (-145, 35)
  line L6 (-95, 35) -> (-45, 35)
  line L7 (-145, 35) -> (-145, 0)
  line L8 (-45, 35) -> (-45, 0)
  line L9 (-45, 0) -> (-145, 0)
  dimension "d152" = 50
  dimension "d153" = 50
  dimension "d154" = 30
  constraint midpoint L3 L4.start
  constraint midpoint L1 L4.end
  constraint coincident L4 L5.start
  constraint perpendicular L4 L5
  constraint perpendicular L4 L6
  constraint coincident L1 L7.end
  constraint perpendicular L1 L7
  constraint coincident L1 L8.end
  constraint perpendicular L1 L8
  measures "d152" distance of L5.start L5.end
  measures "d153" distance of L5.start L6.end
  measures "d154" distance of L3 L5
extrude "Extrude24" add sketch "Sketch20" along normal blind 35 contours L1 L5 L6 L7 L8 L9 bodies 2 in component "Solder Reflow Hot Plate Base"
sketch "Sketch22" plane through (0, 205, 0) normal (0, -1, 0) x (1, 0, 0) in component "Solder Reflow Hot Plate Base"
  line L0 (175, 38.2) -> (15, 38.2)
  line L1 (15, 38.2) -> (15, 14)
  line L2 (15, 14) -> (25, 14)
  line L3 (25, 14) -> (25, 2)
  line L4 (25, 2) -> (15, 2)
  line L5 (15, 2) -> (15, 0)
  line L6 (15, 0) -> (175, 0)
  line L7 (175, 0) -> (175, 2)
  line L8 (175, 2) -> (165, 2)
  line L9 (165, 2) -> (165, 14)
  line L10 (165, 14) -> (175, 14)
  line L11 (175, 14) -> (175, 38.2)
  line L12 (15, 65) -> (175, 65)
  circle A0 centre (95, 18) radius 10
  line L13 (45, 0) -> (15, 0)
  line L14 (95, 65) -> (95, 0) construction
  line L15 (45, 0) -> (145, 0)
  line L16 (175, 0) -> (145, 0)
  dimension "d157" = 20
  dimension "d163" = 18
  constraint midpoint L12 L14.start
  constraint midpoint L6 L14.end
  constraint coincident A0.centre L14
  measures "d157" diameter of A0
  measures "d163" distance of A0.centre L15
extrude "Extrude23" cut sketch "Sketch22" against normal up to surface (5 mm away) contours A0 bodies 2 in component "Solder Reflow Hot Plate Base"
sketch "Sketch23" plane through (45, 0, 0) normal (-1, 0, 0) x (0, -1, 0) in component "Solder Reflow Hot Plate Base"
  line L0 (-210, 0) -> (-210, 35)
  line L1 (-210, 35) -> (-245, 35)
  line L2 (-245, 35) -> (-245, 0)
  line L3 (-245, 0) -> (-210, 0) construction
  line L4 (-245, 0) -> (-245, 3) construction
  line L5 (-245, 3) -> (-213, 35)
  line L6 (-245, 3) -> (-199.7452, 3) construction
  line L7 (-213, 35) -> (-210, 35)
  line L8 (-245, 3) -> (-245, 35)
  line L9 (-213, 35) -> (-245, 35)
  dimension "d164" = 3
  dimension "d165" = 45
  constraint coincident L2.end L3.start
  constraint perpendicular L3 L4
  constraint horizontal L6
  constraint coincident L1 L5.end
  constraint coincident L0.end L1.start
  constraint coincident L1.end L2.start
  measures "d164" distance of L2.end L4.end
  measures "d165" angle of L5 L6
extrude "Extrude25" cut sketch "Sketch23" against normal up to surface (100 mm away) bodies 2 in component "Solder Reflow Hot Plate Base"
fillet "Fillet3" radius 3 2 edges at (95, 213, 35) (95, 245, 3) on bodies 2 in component "Solder Reflow Hot Plate Base"
fillet "Fillet4" radius 3 10 edges at (45, 210.8787, 35) (45, 212.9054, 34.7716) (45, 229, 19) (45, 244.7716, 2.9054) (45, 245, 0.8787) (145, 245, 0.8787) (145, 244.7716, 2.9054) (145, 229, 19) (145, 212.9054, 34.7716) (145, 210.8787, 35) on bodies 2 in component "Solder Reflow Hot Plate Base"
ref_plane "WorkPlane7" through (95, 210, 32.5) normal (0, 1, 0) x (-1, 0, 0) in component "Solder Reflow Hot Plate Base"
split "Split3" by plane through (95, 210, 32.5) normal (0, 1, 0) bodies 2 makes body 3 at (110.6667, 234.0404, 13.9596) in component "Solder Reflow Hot Plate Base"
shell "Shell2" thickness 2 removed faces 2 at (58.3333, 210, 16.6667) at (98.1852, 210, 18.9825) on bodies 3 in component "Solder Reflow Hot Plate Base"
sketch "Sketch24" plane through (0, 210, 0) normal (0, -1, 0) x (1, 0, 0) in component "Solder Reflow Hot Plate Base"
  arc A0 (143, 32) -> (142, 33) centre (142, 32) ccw
  line L0 (143, 32) -> (143, 2)
  line L1 (143, 2) -> (47, 2)
  line L2 (47, 2) -> (47, 32)
  arc A1 (48, 33) -> (47, 32) centre (48, 32) ccw
  line L3 (48, 33) -> (142, 33)
  line L4 (45, 32) -> (45, 0)
  line L5 (45, 0) -> (145, 0)
  line L6 (145, 0) -> (145, 32)
  arc A2 (145, 32) -> (142, 35) centre (142, 32) ccw
  line L7 (142, 35) -> (48, 35)
  arc A3 (48, 35) -> (45, 32) centre (48, 32) ccw
  line L8 (45, 32) -> (45, 0)
  line L9 (45, 0) -> (38.8, 0)
  line L10 (38.8, 0) -> (38.8, 32)
  line L11 (38.8, 32) -> (45, 32)
  line L12 (145, 0) -> (145, 32)
  line L13 (145, 0) -> (151.2, 0)
  line L14 (151.2, 0) -> (151.2, 32)
  line L15 (151.2, 32) -> (145, 32)
  line L16 (148.1, 32) -> (148.1, 0) construction
  line L17 (41.9, 32) -> (41.9, 0) construction
  circle A4 centre (148.1, 29) radius 1.9
  circle A5 centre (148.1, 3) radius 1.9
  circle A6 centre (41.9, 29) radius 1.9
  circle A7 centre (41.9, 3) radius 1.9
  dimension "d174" = 6.2
  dimension "d175" = 6.2
  dimension "d178" = 3.8
  dimension "d179" = 3
  dimension "d180" = 3.8
  dimension "d181" = 3
  dimension "d182" = 3.8
  dimension "d183" = 3.8
  dimension "d184" = 3
  dimension "d185" = 3
  constraint coincident L4.start A3.end
  constraint coincident L4.end L5.start
  constraint perpendicular L8 L9
  constraint perpendicular L9 L10
  constraint perpendicular L4 L11
  constraint coincident L5.end L6.start
  constraint coincident L6.end A2.start
  constraint perpendicular L12 L13
  constraint perpendicular L13 L14
  constraint perpendicular L12 L15
  constraint midpoint L15 L16.start
  constraint midpoint L13 L16.end
  constraint midpoint L11 L17.start
  constraint midpoint L9 L17.end
  constraint coincident L16 A4.centre
  constraint coincident L16 A5.centre
  constraint coincident L17 A6.centre
  constraint coincident L17 A7.centre
  measures "d174" distance of L4.end L9.end
  measures "d175" distance of L5.end L13.end
  measures "d178" diameter of A4
  measures "d179" distance of L15 A4.centre
  measures "d180" diameter of A5
  measures "d181" distance of L13 A5.centre
  measures "d182" diameter of A6
  measures "d183" diameter of A7
  measures "d184" distance of L11 A6.centre
  measures "d185" distance of L9 A7.centre
extrude "Extrude26" add sketch "Sketch24" against normal blind 2 contours L4 L8 L9 L10 L11 | L6 L12 L13 L14 L15 bodies 3 in component "Solder Reflow Hot Plate Base"
fillet "Fillet5" radius 3 4 edges at (38.8, 211, 32) (38.8, 211, 0) (151.2, 211, 32) (151.2, 211, 0) on bodies 3 in component "Solder Reflow Hot Plate Base"
sketch "Sketch25" plane through (0, 210, 0) normal (0, 1, 0) x (-1, 0, 0) in component "Solder Reflow Hot Plate Base"
  circle A0 centre (-95, 18) radius 10
  line L0 (-175, 0) -> (-15, 0)
  line L1 (-15, 0) -> (-15, 65)
  line L2 (-15, 65) -> (-175, 65)
  line L3 (-175, 65) -> (-175, 0)
  circle A1 centre (-41.9, 29) radius 1.9
  circle A2 centre (-41.9, 3) radius 1.9
  circle A3 centre (-148.1, 29) radius 1.9
  circle A4 centre (-148.1, 3) radius 1.9
  circle A5 centre (-41.9, 29) radius 2.05
  circle A6 centre (-41.9, 3) radius 2.05
  circle A7 centre (-148.1, 29) radius 2.05
  circle A8 centre (-148.1, 3) radius 2.05
  dimension "d188" = 4.1
  dimension "d189" = 4.1
  dimension "d190" = 4.1
  dimension "d191" = 4.1
  constraint concentric A1 A5
  constraint concentric A2 A6
  constraint concentric A3 A7
  constraint concentric A4 A8
  measures "d188" diameter of A5
  measures "d189" diameter of A6
  measures "d190" diameter of A7
  measures "d191" diameter of A8
extrude "Extrude27" cut sketch "Sketch25" against normal up to surface (5 mm away) contours A1 | A2 | A3 | A4 | A5 | A6 | A7 | A8 bodies 2 in component "Solder Reflow Hot Plate Base"
sketch "Sketch26" plane through (0, 124, 124) normal (0, 0.707107, 0.707107) x (-1, 0, 0) in component "Solder Reflow Hot Plate Base"
  line L0 (-142, -127.1076) -> (-142, -169.8772)
  line L1 (-142, -169.8772) -> (-48, -169.8772)
  line L2 (-48, -169.8772) -> (-48, -127.1076)
  line L3 (-48, -127.1076) -> (-142, -127.1076)
  line L4 (-142, -148.4924) -> (-48, -148.4924) construction
  line L5 (-96.5, -136.7424) -> (-131.5, -136.7424)
  line L6 (-131.5, -136.7424) -> (-131.5, -160.2424)
  line L7 (-131.5, -160.2424) -> (-96.5, -160.2424)
  line L8 (-96.5, -160.2424) -> (-96.5, -136.7424)
  line L9 (-96.5, -136.7424) -> (-131.5, -160.2424) construction
  line L10 (-131.5, -136.7424) -> (-96.5, -160.2424) construction
  line L11 (-68, -127.1076) -> (-68, -169.8772) construction
  circle A0 centre (-68, -148.4924) radius 4
  circle A1 centre (-68, -148.4924) radius 7.5 construction
  point P0 (-114, -148.4924)
  dimension "d198" = 35
  dimension "d199" = 23.5
  dimension "d200" = 28
  dimension "d201" = 20
  dimension "d202" = 8
  dimension "d203" = 15
  constraint midpoint L0 L4.start
  constraint midpoint L2 L4.end
  constraint horizontal L5
  constraint perpendicular L5 L6
  constraint parallel L5 L7
  constraint parallel L6 L8
  constraint coincident L9 P0
  constraint coincident L10 P0
  constraint coincident L4 P0
  constraint coincident L3 L11.start
  constraint coincident L1 L11.end
  constraint perpendicular L1 L11
  constraint midpoint L11 A0.centre
  constraint concentric A0 A1
  measures "d198" distance of L6.end L7.end
  measures "d199" distance of L5.end L6.end
  measures "d200" distance of L0 P0
  measures "d201" distance of L2 L11
  measures "d202" diameter of A0
  measures "d203" diameter of A1
extrude "Extrude28" cut sketch "Sketch26" against normal up to surface (2 mm away) contours L5 L6 L7 L8 | A0 bodies 3 in component "Solder Reflow Hot Plate Base"